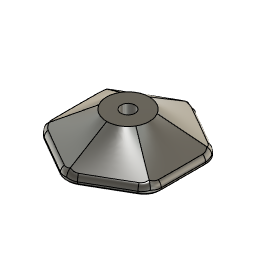
Mounting Plate Parametric (Autodesk Fusion 360 design; units mm, degrees)
Autodesk Fusion 360 part; units mm, degrees
sketch "Sketch1" plane through (0, 0, 0) normal (0, 0, 1) x (1, 0, 0) in component "Mounting Plate"
  line L0 (0, 37.5278) -> (-32.5, 18.7639)
  line L1 (-32.5, 18.7639) -> (-32.5, -18.7639)
  line L2 (-32.5, -18.7639) -> (0, -37.5278)
  line L3 (0, -37.5278) -> (32.5, -18.7639)
  line L4 (32.5, -18.7639) -> (32.5, 18.7639)
  line L5 (32.5, 18.7639) -> (0, 37.5278)
  circle A0 centre (0, 0) radius 3.8735 construction
  circle A1 centre (0, 0) radius 4.1735
  circle A2 centre (0, 0) radius 8.25 construction
  line L6 (9.75, 0.375) -> (6.75, 0.375)
  line L7 (6.75, 0.375) -> (6.75, -0.375)
  line L8 (6.75, -0.375) -> (9.75, -0.375)
  line L9 (9.75, -0.375) -> (9.75, 0.375)
  line L10 (9.75, 0.375) -> (6.75, -0.375) construction
  line L11 (6.75, 0.375) -> (9.75, -0.375) construction
  line L12 (10.025, -5.7879) -> (10.025, 5.7879) construction
  line L13 (10.025, 5.7879) -> (0, 11.5759) construction
  line L14 (0, 11.5759) -> (-10.025, 5.7879) construction
  line L15 (-10.025, 5.7879) -> (-10.025, -5.7879) construction
  line L16 (-10.025, -5.7879) -> (0, -11.5759) construction
  line L17 (0, -11.5759) -> (10.025, -5.7879) construction
  line L18 (-10.325, 5.9611) -> (-10.325, -5.9611)
  line L19 (-10.325, -5.9611) -> (0, -11.9223)
  line L20 (0, -11.9223) -> (10.325, -5.9611)
  line L21 (10.325, -5.9611) -> (10.325, 5.9611)
  line L22 (10.325, 5.9611) -> (0, 11.9223)
  line L23 (0, 11.9223) -> (-10.325, 5.9611)
  point P0 (8.25, 0)
  dimension "d1" = 65
  dimension "d11" = 7.747
  dimension "d13" = 0.3
  dimension "d20" = 16.5
  dimension "d21" = 0.75
  dimension "d22" = 3
  dimension "d35" = 20.05
  dimension "d36" = 0.3
  constraint coincident A0.centre A1.centre
  constraint vertical L4
  constraint horizontal L6
  constraint perpendicular L6 L7
  constraint parallel L6 L8
  constraint parallel L7 L9
  constraint coincident L10 P0
  constraint coincident L11 P0
  constraint coincident A2 P0
  constraint vertical L12
  constraint horizontal A0.centre P0
  measures "d1" distance of L1 L4
  measures "d11" diameter of A0
  measures "d20" diameter of A2
  measures "d21" distance of L6.end L7.end
  measures "d22" distance of L7.end L8.end
  measures "d35" distance of L12 L15
ref_plane "WorkPlane1" through (0, 0, 15.1125) normal (0, 0, 1) x (1, 0, 0) in component "Mounting Plate"
sketch "Sketch2" plane through (0, 0, 15.1125) normal (0, 0, 1) x (1, 0, 0) in component "Mounting Plate"
  circle A0 centre (0, 0) radius 12.5
  dimension "d9" = 25
  constraint coincident A0.centre origin
  measures "d9" diameter of A0
loft "Loft1" add profiles "Sketch1", "Sketch2" section 1 contours L0 L1 L2 L3 L4 L5 | A1 | L6 L7 L8 L9 | L18 L19 L20 L21 L22 L23 section 2 makes body 1 in component "Mounting Plate"
extrude "Extrude1" cut sketch "Sketch1" along normal blind 20 and the other way blind 20 contours A1 bodies 1 in component "Mounting Plate"
extrude "Extrude2" add sketch "Sketch1" against normal blind 4 contours L0 L1 L2 L3 L4 L5 bodies 1 in component "Mounting Plate"
extrude "Extrude8" cut 1 faces at (-4.1373, -7.1659, 0) along direction (0, 0, 1) blind 4 on bodies 1 bodies 1 in component "Mounting Plate"
extrude "Extrude3" cut sketch "Sketch1" along normal blind 10 contours L6 L7 L8 L9 bodies 1 in component "Mounting Plate"
pattern_circular "C-Pattern1" count 12 over 360 about axis through (0, 0, 0) along (0, 0, 1) of "Extrude3" in component "Mounting Plate"
sketch "Sketch3" plane through (0, 0, 4) normal (0, 0, 1) x (1, 0, 0) in component "Mounting Plate"
  line L0 (0, -11.9223) -> (10.325, -5.9611)
  line L1 (10.325, -5.9611) -> (10.325, 5.9611)
  line L2 (10.325, 5.9611) -> (0, 11.9223)
  line L3 (0, 11.9223) -> (-10.325, 5.9611)
  line L4 (-10.325, 5.9611) -> (-10.325, -5.9611)
  line L5 (-10.325, -5.9611) -> (0, -11.9223)
  line L6 (5.6582, -3.6998) -> (8.2562, -5.1998)
  line L7 (8.2562, -5.1998) -> (8.6312, -4.5502)
  line L8 (8.6312, -4.5502) -> (6.0332, -3.0502)
  line L9 (6.0332, -3.0502) -> (5.6582, -3.6998)
  line L10 (3.0502, -6.0332) -> (4.5502, -8.6312)
  line L11 (4.5502, -8.6312) -> (5.1998, -8.2562)
  line L12 (5.1998, -8.2562) -> (3.6998, -5.6582)
  line L13 (3.6998, -5.6582) -> (3.0502, -6.0332)
  line L14 (-0.375, -6.75) -> (-0.375, -9.75)
  line L15 (-0.375, -9.75) -> (0.375, -9.75)
  line L16 (0.375, -9.75) -> (0.375, -6.75)
  line L17 (0.375, -6.75) -> (-0.375, -6.75)
  line L18 (-3.6998, -5.6582) -> (-5.1998, -8.2562)
  line L19 (-5.1998, -8.2562) -> (-4.5502, -8.6312)
  line L20 (-4.5502, -8.6312) -> (-3.0502, -6.0332)
  line L21 (-3.0502, -6.0332) -> (-3.6998, -5.6582)
  line L22 (-6.0332, -3.0502) -> (-8.6312, -4.5502)
  line L23 (-8.6312, -4.5502) -> (-8.2562, -5.1998)
  line L24 (-8.2562, -5.1998) -> (-5.6582, -3.6998)
  line L25 (-5.6582, -3.6998) -> (-6.0332, -3.0502)
  line L26 (-6.75, 0.375) -> (-9.75, 0.375)
  line L27 (-9.75, 0.375) -> (-9.75, -0.375)
  line L28 (-9.75, -0.375) -> (-6.75, -0.375)
  line L29 (-6.75, -0.375) -> (-6.75, 0.375)
  line L30 (-5.6582, 3.6998) -> (-8.2562, 5.1998)
  line L31 (-8.2562, 5.1998) -> (-8.6312, 4.5502)
  line L32 (-8.6312, 4.5502) -> (-6.0332, 3.0502)
  line L33 (-6.0332, 3.0502) -> (-5.6582, 3.6998)
  line L34 (-3.0502, 6.0332) -> (-4.5502, 8.6312)
  line L35 (-4.5502, 8.6312) -> (-5.1998, 8.2562)
  line L36 (-5.1998, 8.2562) -> (-3.6998, 5.6582)
  line L37 (-3.6998, 5.6582) -> (-3.0502, 6.0332)
  line L38 (0.375, 6.75) -> (0.375, 9.75)
  line L39 (0.375, 9.75) -> (-0.375, 9.75)
  line L40 (-0.375, 9.75) -> (-0.375, 6.75)
  line L41 (-0.375, 6.75) -> (0.375, 6.75)
  line L42 (3.6998, 5.6582) -> (5.1998, 8.2562)
  line L43 (5.1998, 8.2562) -> (4.5502, 8.6312)
  line L44 (4.5502, 8.6312) -> (3.0502, 6.0332)
  line L45 (3.0502, 6.0332) -> (3.6998, 5.6582)
  line L46 (6.0332, 3.0502) -> (8.6312, 4.5502)
  line L47 (8.6312, 4.5502) -> (8.2562, 5.1998)
  line L48 (8.2562, 5.1998) -> (5.6582, 3.6998)
  line L49 (5.6582, 3.6998) -> (6.0332, 3.0502)
  line L50 (6.75, -0.375) -> (9.75, -0.375)
  line L51 (9.75, -0.375) -> (9.75, 0.375)
  line L52 (9.75, 0.375) -> (6.75, 0.375)
  line L53 (6.75, 0.375) -> (6.75, -0.375)
  line L54 (0, 11.9223) -> (10.325, 5.9611)
  line L55 (10.325, 5.9611) -> (10.325, -5.9611)
  line L56 (10.325, -5.9611) -> (0, -11.9223)
  line L57 (0, -11.9223) -> (-10.325, -5.9611)
  line L58 (-10.325, -5.9611) -> (-10.325, 5.9611)
  line L59 (-10.325, 5.9611) -> (0, 11.9223)
  circle A0 centre (0, 0) radius 4.1735
  point P0 (0, -11.9223)
  constraint coincident A0.centre origin
  constraint coincident P0 L0.start
extrude "Extrude4" add sketch "Sketch3" against normal blind 0.2 separate body contours L0 L1 L2 L3 L4 L5 L54 L55 L56 L57 L58 L59 | L6 L7 L8 L9 | L10 L11 L12 L13 | L14 L15 L16 L17 | L18 L19 L20 L21 | L22 L23 L24 L25 | L26 L27 L28 L29 | L30 L31 L32 L33 | L34 L35 L36 L37 | L38 L39 L40 L41 | L42 L43 L44 L45 | L46 L47 L48 L49 | L50 L51 L52 L53 | A0 makes body 2 in component "Mounting Plate"
fillet "Fillet1" radius 10 6 edges at (32.5, 18.7639, -2) (32.5, -18.7639, -2) (0, 37.5278, -2) (-32.5, 18.7639, -2) (-32.5, -18.7639, -2) (0, -37.5278, -2) on bodies 1 in component "Mounting Plate"
fillet "Fillet2" radius 4 18 edges at (-32.1494, 15.6153, 0.25) (-32.5, 0, 0) (-32.1499, -15.6132, 0.2496) (2.5514, -35.6498, 0.25) (16.25, -28.1458, 0) (29.5964, -20.0361, 0.2496) (32.1494, -15.6153, 0.25) (32.5, 0, 0) (32.1499, 15.6132, 0.2496) (29.598, 20.0345, 0.25) (16.25, 28.1458, 0) (2.5536, 35.6492, 0.2496) (-2.5514, 35.6498, 0.25) (-16.25, 28.1458, 0) (-29.5964, 20.0361, 0.2496) (-29.598, -20.0345, 0.25) (-16.25, -28.1458, 0) (-2.5536, -35.6492, 0.2496) on bodies 1 in component "Mounting Plate"
chamfer "Chamfer1" distance 1 angle 45 12 edges at (0, 35.9808, -4) (-16.25, 28.1458, -4) (-31.1603, 17.9904, -4) (-32.5, 0, -4) (-31.1603, -17.9904, -4) (-16.25, -28.1458, -4) (0, -35.9808, -4) (16.25, -28.1458, -4) (31.1603, -17.9904, -4) (32.5, 0, -4) (31.1603, 17.9904, -4) (16.25, 28.1458, -4) on bodies 1 in component "Mounting Plate"
sketch "Sketch1 (2)" plane through (0, 0, -4) normal (0, 0, -1) x (1, 0, 0) in component "T Nut Cover"
  arc A0 (-4.5, -33.775) -> (4.5, -33.775) centre (0, -25.9808) ccw
  line L0 (4.5, -33.775) -> (27, -20.7846)
  arc A1 (27, -20.7846) -> (31.5, -12.9904) centre (22.5, -12.9904) ccw
  line L1 (31.5, -12.9904) -> (31.5, 12.9904)
  arc A2 (31.5, 12.9904) -> (27, 20.7846) centre (22.5, 12.9904) ccw
  line L2 (27, 20.7846) -> (4.5, 33.775)
  arc A3 (4.5, 33.775) -> (-4.5, 33.775) centre (0, 25.9808) ccw
  line L3 (-4.5, 33.775) -> (-27, 20.7846)
  arc A4 (-27, 20.7846) -> (-31.5, 12.9904) centre (-22.5, 12.9904) ccw
  line L4 (-31.5, 12.9904) -> (-31.5, -12.9904)
  arc A5 (-31.5, -12.9904) -> (-27, -20.7846) centre (-22.5, -12.9904) ccw
  line L5 (-27, -20.7846) -> (-4.5, -33.775)
  line L6 (0, -11.9223) -> (-10.325, -5.9611)
  line L7 (-10.325, -5.9611) -> (-10.325, 5.9611)
  line L8 (-10.325, 5.9611) -> (0, 11.9223)
  line L9 (0, 11.9223) -> (10.325, 5.9611)
  line L10 (10.325, 5.9611) -> (10.325, -5.9611)
  line L11 (10.325, -5.9611) -> (0, -11.9223)
  line L12 (10.025, -5.7879) -> (0, -11.5759)
  line L13 (0, -11.5759) -> (-10.025, -5.7879)
  line L14 (-10.025, -5.7879) -> (-10.025, 5.7879)
  line L15 (-10.025, 5.7879) -> (0, 11.5759)
  line L16 (0, 11.5759) -> (10.025, 5.7879)
  line L17 (10.025, 5.7879) -> (10.025, -5.7879)
  dimension "d81" = 0.3
extrude "Extrude1'" add sketch "Sketch1 (2)" against normal blind 5.5 separate body contours L12 L13 L14 L15 L16 L17 makes body 3 in component "T Nut Cover"
sketch "Sketch2 (2)" plane through (0, 0, 1.5) normal (0, 0, 1) x (-1, 0, 0) in component "T Nut Cover"
  line L0 (0, 11.5759) -> (-10.025, 5.7879)
  line L1 (-10.025, 5.7879) -> (-10.025, -5.7879)
  line L2 (-10.025, -5.7879) -> (0, -11.5759)
  line L3 (0, -11.5759) -> (10.025, -5.7879)
  line L4 (10.025, -5.7879) -> (10.025, 5.7879)
  line L5 (10.025, 5.7879) -> (0, 11.5759)
  circle A0 centre (0, 0) radius 5
  dimension "d104" = 10
  constraint coincident A0.centre origin
  measures "d104" diameter of A0
extrude "Extrude2'" cut sketch "Sketch2 (2)" against normal blind 3 contours A0 bodies 3 in component "T Nut Cover"
sketch "Sketch7" plane through (0, 0, 0) normal (0, 1, 0) x (1, 0, 0) in component "Mounting Plate"
  line L0 (9.75, -4) -> (9.75, -10)
  line L1 (10.325, -1.5) -> (11.325, -1.5) construction
  line L2 (4.5, 4) -> (27, 4) construction
  line L3 (11.325, 4) -> (11.325, -1.5) construction
  line L4 (6.75, -4) -> (9.75, -4) construction
  line L5 (10.325, 4) -> (10.325, -4) construction
  line L6 (11.325, 1.25) -> (10.325, 2.25)
  line L7 (11.325, 1.25) -> (10.325, 1.25) construction
  line L8 (11.325, 1.25) -> (10.325, 0.25)
  line L9 (11.325, 1.25) -> (10.325, 1.25) construction
  line L10 (10.325, 2.25) -> (10.325, 0.25)
  point P0 (10.325, -4)
  dimension "d96" = 1
  dimension "d97" = 45
  dimension "d98" = 45
  dimension "d112" = 5.5
  constraint coincident L2 L3.start
  constraint horizontal L1
  constraint vertical L3
  constraint horizontal L7
  constraint midpoint L3 L6.start
  constraint coincident L5 L6.end
  constraint horizontal L9
  constraint coincident L5 L8.end
  constraint coincident L1.start L5
  constraint midpoint L7.end L10
  measures "d96" distance of L3 L5
  measures "d97" angle of L6 L7
  measures "d98" angle of L8 L9
  measures "d112" distance of L1.start L5.start
extrude "Extrude9" cut sketch "Sketch7" along normal blind 2 and the other way blind 2 bodies 1 in component "Mounting Plate"
pattern_circular "C-Pattern2" count 6 over 360 about axis through (0, 0, 4) along (0, 0, -1) of "Extrude9" in component "Mounting Plate"
sketch "Sketch4" plane through (0, 0, 0) normal (0, 1, 0) x (1, 0, 0) in component "T Nut Cover"
  line L0 (-10.025, 4) -> (-10.025, -1.5)
  line L1 (-10.025, 0.25) -> (-11.025, 1.25)
  line L2 (-10.025, 2.25) -> (-11.025, 1.25)
  line L3 (-11.025, 1.25) -> (-10.025, 1.25) construction
  dimension "d107" = 1
  dimension "d113" = 45
  dimension "d114" = 45
  constraint coincident L0 L1.start
  constraint coincident L0 L2.start
  constraint midpoint L0 L3.end
  constraint horizontal L3
  measures "d107" distance of L0 L1.end
  measures "d113" angle of L2 L3
  measures "d114" angle of L1 L3
extrude "Extrude3'" add sketch "Sketch4" along normal blind 1.7 and the other way blind 1.7 bodies 3 in component "T Nut Cover"
fillet "Fillet2'" radius 1 1 edges at (-11.025, 0, -1.25) on bodies 3 in component "T Nut Cover"
pattern_circular "C-Pattern1'" count 6 over 360 about axis through (0, 0, 1.75) along (0, 0, 1) of "Extrude3'", "Fillet2'" in component "T Nut Cover"
chamfer "Chamfer1'" distance 1 angle 45 1 faces at (-4.175, -7.2313, 1.5) on bodies 3 in component "T Nut Cover"
sketch "Sketch8" plane through (0, 0, -4) normal (0, 0, -1) x (1, 0, 0) in component "Mounting Plate"
  line L0 (10.325, -5.9611) -> (0, -11.9223)
  line L1 (0, -11.9223) -> (-10.325, -5.9611)
  line L2 (-10.325, -5.9611) -> (-10.325, 5.9611)
  line L3 (-10.325, 5.9611) -> (0, 11.9223)
  line L4 (0, 11.9223) -> (10.325, 5.9611)
  line L5 (10.325, 5.9611) -> (10.325, -5.9611)
  arc A0 (-4.5, -33.775) -> (4.5, -33.775) centre (0, -25.9808) ccw
  line L6 (4.5, -33.775) -> (27, -20.7846)
  arc A1 (27, -20.7846) -> (31.5, -12.9904) centre (22.5, -12.9904) ccw
  line L7 (31.5, -12.9904) -> (31.5, 12.9904)
  arc A2 (31.5, 12.9904) -> (27, 20.7846) centre (22.5, 12.9904) ccw
  line L8 (27, 20.7846) -> (4.5, 33.775)
  arc A3 (4.5, 33.775) -> (-4.5, 33.775) centre (0, 25.9808) ccw
  line L9 (-4.5, 33.775) -> (-27, 20.7846)
  arc A4 (-27, 20.7846) -> (-31.5, 12.9904) centre (-22.5, 12.9904) ccw
  line L10 (-31.5, 12.9904) -> (-31.5, -12.9904)
  arc A5 (-31.5, -12.9904) -> (-27, -20.7846) centre (-22.5, -12.9904) ccw
  line L11 (-27, -20.7846) -> (-4.5, -33.775)
  line L12 (11.325, -2) -> (11.325, 2)
  line L13 (11.325, -2) -> (10.325, -2)
  line L14 (10.325, -2) -> (10.325, 2)
  line L15 (10.325, 2) -> (11.325, 2)
  line L16 (11.325, 2) -> (11.325, -2)
  constraint horizontal L13
  constraint vertical L14
  constraint horizontal L15
  constraint vertical L16
  constraint coincident L5 L14.end
  constraint coincident L12.start L13.start
  constraint coincident L12.end L15.end
extrude "Extrude7" cut sketch "Sketch8" against normal blind 5.8062 contours L5 L12 L13 L14 L15 L16 bodies 1 in component "Mounting Plate"
chamfer "Chamfer4" distance 1 angle 45 3 edges at (10.825, -2, -4) (11.325, 0, -4) (10.825, 2, -4) on bodies 1 in component "Mounting Plate"
component "Mounting Plate" placed x (1, 0, 0) y (0, 1, 0) z (0, 0, 1) at (0, 0, 0)
component "T Nut Cover" placed x (1, 0, 0) y (0, 1, 0) z (0, 0, 1) at (0, 0, 0)
equation "d1 = Plate_Width"
equation "Plate_Width = 65 mm"
equation "d8 = Tee_Nut_Barrel_Height + 4 mm"
equation "d11 = Tee_Nut_Barrel_Diameter"
equation "d13 = Tolerance"
equation "d35 = Tee_Nut_Flange_Diameter + 1 mm"
equation "d36 = Tolerance"
equation "d69 = 2 mm - Tolerance"
equation "d76 = -8 mm + Tee_Nut_Flange_Thickness + 1 mm"
equation "Tolerance = 0.3 mm"
equation "d81 = Tolerance"
equation "Tee_Nut_Barrel_Diameter = 0.305 in"
equation "Tee_Nut_Barrel_Height = ( 7 / 16 ) * 1 in"
equation "Tee_Nut_Flange_Diameter = ( 3 / 4 ) * 1 in"
equation "Tee_Nut_Flange_Thickness = 0.047 in"
equation "d108 = 2 mm - Tolerance"
named bodies: "Mounting Plate", "Unsupported Hole"
